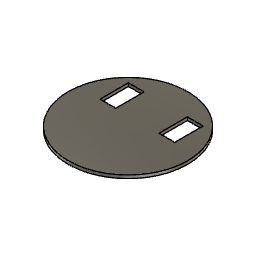
Support robot v2 (Autodesk Fusion 360 design; units mm, degrees)
Autodesk Fusion 360 part; units mm, degrees
sketch "Esquisse1" plane through (0, 0, 0) normal (0, 0, 1) x (1, 0, 0)
  circle A0 centre (0, 0) radius 95
  dimension "d1" = 190
  constraint coincident A0.centre origin
  measures "d1" diameter of A0
extrude "Extrusion1" add sketch "Esquisse1" along normal blind 5
sketch "Esquisse2" plane through (0, 0, 5) normal (0, 0, 1) x (-1, 0, 0)
  circle A0 centre (0, 0) radius 95
  line L0 (-34.3905, -60) -> (-59.3905, -60)
  line L1 (-59.3905, -60) -> (-59.3905, -15)
  line L2 (-59.3905, -15) -> (-34.3905, -15)
  line L3 (-34.3905, -15) -> (-34.3905, -60)
  line L4 (0, 95) -> (0, -95)
  line L5 (34.3905, -15) -> (34.3905, -60)
  line L6 (59.3905, -60) -> (59.3905, -15)
  line L7 (59.3905, -15) -> (34.3905, -15)
  line L8 (34.3905, -60) -> (59.3905, -60)
  dimension "d4" = 25
  dimension "d5" = 45
  constraint horizontal L0
  constraint vertical L1
  constraint horizontal L2
  constraint vertical L3
  constraint coincident A0 L4.start
  constraint coincident A0 L4.end
  constraint vertical L4
  constraint symmetric L0.start L4 L5.end
  constraint symmetric L0.end L4 L6.start
  constraint symmetric L1.end L4 L6.end
  constraint symmetric L2.end L4 L5.start
  measures "d4" distance of L0.start L0.end
  measures "d5" distance of L0.start L2.end
extrude "Extrusion2" cut sketch "Esquisse2" against normal blind 10 contours L0 L1 L2 L3 | L5 L6 L7 L8
